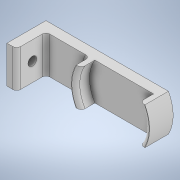
# Autodesk Inventor part: Lid_holder
Saved by Autodesk Inventor 2020 (Build 240168000, 168)
## iProperties
Created: 2023-05-07
Part Number: Lid_holder
Material: Generic
Document SubType Name: Modeling
Designer: DSOB
Density: 1 g/cm^3
Appearance: Default
Author: DSOB
Autodesk Inventor part; units mm, degrees
ref_plane "YZ Plane" through (0, 0, 0) normal (1, 0, 0) x (0, 1, 0)
ref_plane "XZ Plane" through (0, 0, 0) normal (0, 1, 0) x (-1, 0, 0)
ref_plane "XY Plane" through (0, 0, 0) normal (0, 0, 1) x (1, 0, 0)
sketch "Sketch1" plane through (0, 0, 0) normal (0, 0, 1) x (1, 0, 0)
  circle A0 centre (0, 0) radius 17.75
  circle A1 centre (0, 0) radius 20
  dimension "d0" = 35.5
  dimension "d1" = 40
  constraints: 2 centre point, 2 coincident
  measures "d0" diameter of A0
  measures "d1" diameter of A1
extrude "Extrusion1" add sketch "Sketch1" along normal blind 7
sketch "Sketch2" plane through (0, 0, 0) normal (0, 0, -1) x (-1, 0, 0)
  circle A0 centre (0, 0) radius 20 projected
extrude "Extrusion2" add sketch "Sketch2" along normal blind 5
sketch "Sketch3" plane through (0, 0, -5) normal (0, 0, -1) x (-1, 0, 0)
  circle A0 centre (0, 0) radius 20 projected
  line L0 (-17.5997, 9.5) -> (17.5997, 9.5)
  line L1 (-17.5997, -9.5) -> (17.5997, -9.5)
  circle A1 centre (0, 0) radius 20 projected
  line L2 (58, 0) -> (-33, 0) projected
  dimension "d6" = 19
  dimension "d7" = 9.5
  constraints: 4 end point, 4 point on circle, 1 horizontal, 1 parallel
  measures "d6" distance between parallel lines of L1 L0
  measures "d7" distance between parallel lines of L0 L2
extrude "Extrusion3" cut sketch "Sketch3" against normal through all contours L0 A0 | A0 L1
sketch "Sketch4" plane through (0, 0, -5) normal (0, 0, -1) x (-1, 0, 0)
  arc A0 (17.5997, -9.5) -> (17.5997, 9.5) centre (0, 0) ccw projected
  line L0 (17.5997, 9.5) -> (45, 9.5)
  line L1 (45, 9.5) -> (45, -9.5)
  arc A1 (17.5997, -9.5) -> (17.5997, 9.5) centre (0, 0) ccw projected
  line L2 (45, -9.5) -> (17.5997, -9.5)
  line L3 (14.9937, -9.5) -> (-14.9937, -9.5) projected
  arc A2 (-14.9937, 9.5) -> (-14.9937, -9.5) centre (0, 0) ccw projected
  line L4 (-14.9937, 9.5) -> (14.9937, 9.5) projected
  arc A3 (14.9937, -9.5) -> (14.9937, 9.5) centre (0, 0) ccw projected
  dimension "d10" = 90
  dimension "d11" = 45
  constraints: 6 end point, 1 horizontal, 1 perpendicular
  measures "d10" angle of L2 L1
  measures "d11" distance from line of L1 point (0, 0)
extrude "Extrusion4" add sketch "Sketch4" against normal blind 5 contours A0 L0 L1 L2
sketch "Sketch5" plane through (0, 0, 0) normal (0, 0, 1) x (1, 0, 0)
  line L0 (17.5997, -9.5) -> (-45, -9.5) projected
  line L1 (-45, 9.5) -> (17.5997, 9.5) projected
  line L2 (-45, -9.5) -> (-40, -9.5)
  line L3 (-40, -9.5) -> (-40, 9.5)
  line L4 (-40, 9.5) -> (-45, 9.5)
  line L5 (-45, 9.5) -> (-45, -9.5)
  point P0 (0, 0)
  dimension "d14" = 5
  constraints: 8 end point, 2 parallel, 1 horizontal, 1 perpendicular, 1 point on line
  measures "d14" distance between parallel lines of L5 L3
extrude "Extrusion5" add sketch "Sketch5" along normal blind 15
sketch "Sketch6" plane through (-40, -9.5, 0) normal (1, 0, 0) x (0, 0, -1)
  point P0 (0, 9.5)
sketch "Sketch7" plane through (-45, -9.5, -5) normal (-1, 0, 0) x (0, 0, 1)
  line L0 (12, 19) -> (12, 0) projected
  circle A0 centre (12, 9.5) radius 2.25
  point P0 (5, 9.5)
  dimension "d17" = 4.5
  constraints: 1 centre point, 1 midpoint
  measures "d17" diameter of A0
extrude "Extrusion6" cut sketch "Sketch7" against normal up to surface (5 mm away)
fillet "Fillet1" radius 2 1 edges at (-40, 0, 0)
fillet "Fillet2" radius 2 1 edges at (-40, 0, 15)
fillet "Fillet3" radius 2 2 edges at (-17.75, 0, 7) (17.75, 0, 7)
fillet_without_effect "Fillet4"
fillet "Fillet6" radius 2 1 edges at (-20, 0, 0)
body "Solid1"
